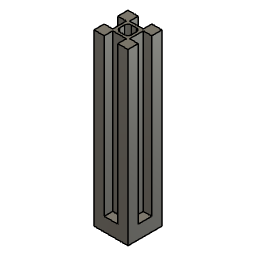
pillar 1cm (Autodesk Fusion 360 design; units mm, degrees)
Autodesk Fusion 360 part; units mm, degrees
sketch "Esquisse1" plane through (0, 0, 0) normal (0, 1, 0) x (1, 0, 0)
  line L0 (30, -20) -> (20, -20)
  line L1 (20, -20) -> (20, -10)
  line L2 (20, -10) -> (30, -10)
  line L3 (30, -10) -> (30, -20)
  circle A0 centre (25, -15) radius 1.25
  dimension "d1" = 10
  dimension "d2" = 10
  dimension "d22" = 2.5
  constraint horizontal L0
  constraint vertical L1
  constraint horizontal L2
  constraint vertical L3
  measures "d1" distance of L0.start L0.end
  measures "d2" distance of L0.start L2.end
  measures "d22" diameter of A0
extrude "Extrusion3" add sketch "Esquisse1" along normal blind 4
sketch "Esquisse3" plane through (0, 4, 0) normal (0, 1, 0) x (-1, 0, 0)
  circle A0 centre (-25, 15) radius 1.25
  line L0 (-30, 10) -> (-20, 10)
  line L1 (-20, 10) -> (-20, 20)
  line L2 (-20, 20) -> (-30, 20)
  line L3 (-30, 20) -> (-30, 10)
  line L4 (-30, 20) -> (-30, 17)
  line L5 (-30, 17) -> (-27.5, 17)
  line L6 (-27.5, 17) -> (-27.5, 15)
  line L7 (-27.5, 15) -> (-27, 15)
  line L8 (-25, 16.75) -> (-25, 17.5)
  line L9 (-25, 17.5) -> (-27, 17.5)
  line L10 (-27, 17.5) -> (-27, 20)
  line L11 (-27, 20) -> (-30, 20)
  line L12 (-30, 17) -> (-30, 20)
  line L13 (-26.75, 15) -> (-27.625, 15)
  line L14 (-25, 17.5) -> (-25, 17)
  line L15 (-25, 16.75) -> (-26.75, 16.75)
  line L16 (-26.75, 16.75) -> (-26.75, 15)
  line L17 (-27.5, 13) -> (-30, 13)
  line L18 (-30, 13) -> (-30, 10)
  line L19 (-30, 10) -> (-27, 10)
  line L20 (-27, 12.5) -> (-25, 12.5)
  line L21 (-25, 12.5) -> (-25, 13)
  line L22 (-27, 10) -> (-27, 12.5)
  line L23 (-25, 13.25) -> (-25, 12.375)
  line L24 (-26.75, 13.25) -> (-25, 13.25)
  line L25 (-26.75, 15) -> (-26.75, 13.25)
  line L26 (-26.75, 15) -> (-27.5, 15)
  line L27 (-27.5, 15) -> (-27.5, 13)
  line L28 (-23, 12.5) -> (-23, 10)
  line L29 (-23, 10) -> (-20, 10)
  line L30 (-20, 10) -> (-20, 13)
  line L31 (-22.5, 13) -> (-22.5, 15)
  line L32 (-22.5, 15) -> (-23, 15)
  line L33 (-20, 13) -> (-22.5, 13)
  line L34 (-23.25, 15) -> (-22.375, 15)
  line L35 (-23.25, 13.25) -> (-23.25, 15)
  line L36 (-25, 13.25) -> (-23.25, 13.25)
  line L37 (-25, 13.25) -> (-25, 12.5)
  line L38 (-25, 12.5) -> (-23, 12.5)
  line L39 (-22.5, 17) -> (-20, 17)
  line L40 (-20, 17) -> (-20, 20)
  line L41 (-20, 20) -> (-23, 20)
  line L42 (-23, 17.5) -> (-25, 17.5)
  line L43 (-25, 17.5) -> (-25, 17)
  line L44 (-23, 20) -> (-23, 17.5)
  line L45 (-25, 16.75) -> (-25, 17.625)
  line L46 (-23.25, 16.75) -> (-25, 16.75)
  line L47 (-23.25, 15) -> (-23.25, 16.75)
  line L48 (-23.25, 15) -> (-22.5, 15)
  line L49 (-22.5, 15) -> (-22.5, 17)
  dimension "d19" = 2.5
  dimension "d20" = 2.5
  dimension "d21" = 2.5
  dimension "d25" = 360
  dimension "d27" = 0.75
  dimension "d28" = 0.75
  dimension "d36" = 4
  dimension "d37" = 3
  dimension "d38" = 3
  dimension "d39" = 3.5
  constraint coincident L2.end L3.start
  constraint coincident L3 L4.end
  constraint perpendicular L2 L4
  constraint perpendicular L4 L5
  constraint perpendicular L5 L6
  constraint perpendicular L6 L7
  constraint perpendicular L8 L9
  constraint coincident L2 L10.end
  constraint perpendicular L2 L10
  constraint perpendicular L2 L12
  constraint perpendicular L8 L15
  constraint perpendicular L13 L16
  measures "d19" distance of L4.end L5.end
  measures "d20" diameter of A0
  measures "d21" distance of L9.end L10.end
  measures "d27" distance of L6 L16
  measures "d28" distance of L9 L15
  measures "d36" distance of L10 L44
  measures "d37" distance of L2.end L10.end
  measures "d38" distance of L2.end L4.end
  measures "d39" distance of L24.start L35.start
extrude "Extrusion6" add sketch "Esquisse3" along normal blind 46 contours L0 L3 L7 L13 L17 L18 L19 L20 L21 L22 L23 L24 L25 L26 L27 L37 | L0 L1 L21 L23 L28 L29 L30 L31 L32 L33 L34 L35 L36 L37 L38 L48 | L2 L3 L4 L5 L6 L7 L8 L9 L10 L11 L12 L13 L14 L15 L16 L26 L43 L45 | L1 L2 L8 L14 L32 L34 L39 L40 L41 L42 L43 L44 L45 L46 L47 L48 L49
fillet "Congé2" radius 1 4 edges at (23.25, 27, 13.25) (26.75, 27, 13.25) (26.75, 27, 16.75) (23.25, 27, 16.75)
sketch "Esquisse4" plane through (0, 0, 0) normal (0, -1, 0) x (1, 0, 0)
  circle A0 centre (25, 15) radius 1.25
  line L0 (20, 10) -> (30, 10)
  line L1 (30, 10) -> (30, 20)
  line L2 (30, 20) -> (20, 20)
  line L3 (20, 20) -> (20, 10)
  line L4 (23.5266, 12.5173) -> (26.4134, 12.4827)
  line L5 (26.4134, 12.4827) -> (27.8868, 14.9654)
  line L6 (27.8868, 14.9654) -> (26.4734, 17.4827)
  line L7 (26.4734, 17.4827) -> (23.5866, 17.5173)
  line L8 (23.5866, 17.5173) -> (20, 17.5173)
  line L9 (23.5266, 12.5173) -> (20, 12.5173)
  point P0 (25, 15)
  constraint coincident L3 L8.end
  constraint perpendicular L3 L8
  constraint coincident L3 L9.end
  constraint perpendicular L3 L9
extrude "Extrusion7" cut sketch "Esquisse4" against normal blind 2 contours L3 L4 L5 L6 L7 L8 L9
